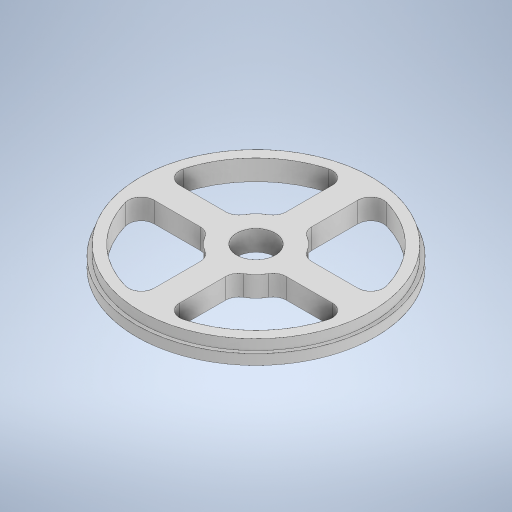
# Autodesk Inventor part: Test_Socle
Saved by Autodesk Inventor 2024 (Build 280153000, 153)
## iProperties
Created: 2025-01-20
Part Number: Test_Socle
Material: Générique
Document SubType Name: Modeling
Designer: malam
Density: 1 g/cm^3
Appearance: Par défaut
Author: malam
Autodesk Inventor part; units mm, degrees
ref_plane "YZ Plane" through (0, 0, 0) normal (1, 0, 0) x (0, 1, 0)
ref_plane "XZ Plane" through (0, 0, 0) normal (0, 1, 0) x (-1, 0, 0)
ref_plane "XY Plane" through (0, 0, 0) normal (0, 0, 1) x (1, 0, 0)
sketch "Esquisse1" plane through (0, 0, 0) normal (0, 1, 0) x (-1, 0, 0)
  circle A0 centre (0, 0) radius 7.5
  circle A1 centre (0, 0) radius 45.155
  circle A2 centre (0, 0) radius 46.595
  dimension "d0" = 15
  dimension "d1" = 90.31
  dimension "d2" = 93.19
  constraints: 3 centre point, 3 coincident
  measures "d0" diameter of A0
  measures "d1" diameter of A1
  measures "d2" diameter of A2
extrude "Extrusion1" add sketch "Esquisse1" along normal blind 4 contours A2
extrude "Extrusion2" add sketch "Esquisse1" along normal blind 8 contours A1
sketch "Esquisse2" plane through (0, 8, 0) normal (0, 1, 0) x (1, 0, 0)
  circle A0 centre (0, 0) radius 45.155 projected
  circle A1 centre (0, 0) radius 7.5 projected
  circle A2 centre (0, 0) radius 14.5
  circle A3 centre (0, 0) radius 41.155
  line L0 (-13.6107, -5) -> (-40.8501, -5)
  line L1 (-14.5, 0) -> (-41.155, 0) construction
  line L2 (-13.6107, 5) -> (-40.8501, 5)
  line L3 (5, -13.6107) -> (5, -40.8501)
  line L4 (-5, -13.6107) -> (-5, -40.8501)
  line L5 (13.6107, 5) -> (40.8501, 5)
  line L6 (13.6107, -5) -> (40.8501, -5)
  line L7 (-5, 13.6107) -> (-5, 40.8501)
  line L8 (5, 13.6107) -> (5, 40.8501)
  dimension "d7" = 7
  dimension "d8" = 4
  dimension "d9" = 5
  dimension "d10" = 5
  dimension "d13" = 360
  constraints: 18 end point, 6 point on circle, 4 horizontal, 2 centre point, 25 other
  measures "d7" radial gap between concentric circles of A1 A2
  measures "d8" radial gap between concentric circles of A0 A3
  measures "d9" distance between parallel lines of L1 L0
  measures "d10" distance between parallel lines of L1 L2
extrude "Extrusion3" cut sketch "Esquisse2" against normal through all contours A2 L8 A3 L5 | L6 A3 L3 A2 | A2 L2 A3 L7 | L4 A3 L0 A2
fillet "Congé1" radius 5 16 edges at (-40.8501, 4, 5) (-5, 4, 40.8501) (5, 4, 40.8501) (-40.8501, 4, -5) (40.8501, 4, 5) (-5, 4, -40.8501) (5, 4, -40.8501) (40.8501, 4, -5) (5, 4, -13.6107) (13.6107, 4, -5) (13.6107, 4, 5) (5, 4, 13.6107) (-5, 4, 13.6107) (-13.6107, 4, 5) (-13.6107, 4, -5) (-5, 4, -13.6107)
